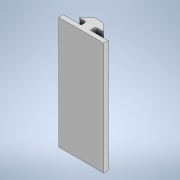
# Autodesk Inventor part: ZItemSpacer
Saved by Autodesk Inventor 2020 (Build 240168000, 168)
## iProperties
Created: 2022-06-06
Part Number: ZItemSpacer
Material: Ogólny
Document SubType Name: Modeling
Designer: mikoma
Density: 1 g/cm^3
Appearance: Domyślna
Author: mikoma
Autodesk Inventor part; units mm, degrees
ref_plane "YZ Plane" through (0, 0, 0) normal (1, 0, 0) x (0, 1, 0)
ref_plane "XZ Plane" through (0, 0, 0) normal (0, 1, 0) x (-1, 0, 0)
ref_plane "XY Plane" through (0, 0, 0) normal (0, 0, 1) x (1, 0, 0)
sketch "Szkic1" plane through (0, 0, 0) normal (0, 1, 0) x (-1, 0, 0)
  arc A0 (11.3, 0) -> (10.5, -0.8) centre (11.3, -0.8) ccw
  line L0 (10.5, -0.8) -> (10.5, -1.5)
  arc A1 (10.5, -1.5) -> (10.8, -1.8) centre (10.8, -1.5) ccw
  line L1 (10.8, -1.8) -> (12.9176, -1.8)
  arc A2 (13.5062, -3.221) -> (12.9176, -1.8) centre (12.9176, -2.6324) ccw
  line L2 (13.5062, -3.221) -> (11.2559, -5.4713)
  arc A3 (9.1346, -6.35) -> (11.2559, -5.4713) centre (9.1346, -3.35) ccw
  line L3 (9.1346, -6.35) -> (6.8654, -6.35)
  arc A4 (4.7441, -5.4713) -> (6.8654, -6.35) centre (6.8654, -3.35) ccw
  line L4 (4.7441, -5.4713) -> (2.4938, -3.221)
  arc A5 (3.0824, -1.8) -> (2.4938, -3.221) centre (3.0824, -2.6324) ccw
  line L5 (3.0824, -1.8) -> (5.2, -1.8)
  arc A6 (5.2, -1.8) -> (5.5, -1.5) centre (5.2, -1.5) ccw
  line L6 (5.5, -1.5) -> (5.5, -0.8)
  arc A7 (5.5, -0.8) -> (4.7, 0) centre (4.7, -0.8) ccw
  line L7 (0, 0) -> (4.7, 0)
  arc A8 (0, 0) -> (-2, -2) centre (0, -2) ccw
  line L8 (-2, -6.7) -> (-2, -2)
  arc A9 (-2, -6.7) -> (-1.2, -7.5) centre (-1.2, -6.7) ccw
  line L9 (-1.2, -7.5) -> (-0.5, -7.5)
  arc A10 (-0.5, -7.5) -> (-0.2, -7.2) centre (-0.5, -7.2) ccw
  line L10 (-0.2, -7.2) -> (-0.2, -5.0824)
  arc A11 (1.221, -4.4938) -> (-0.2, -5.0824) centre (0.6324, -5.0824) ccw
  line L11 (1.221, -4.4938) -> (3.4713, -6.7441)
  arc A12 (4.35, -8.8654) -> (3.4713, -6.7441) centre (1.35, -8.8654) ccw
  line L12 (4.35, -8.8654) -> (4.35, -11.1346)
  arc A13 (3.4713, -13.2559) -> (4.35, -11.1346) centre (1.35, -11.1346) ccw
  line L13 (3.4713, -13.2559) -> (1.221, -15.5062)
  arc A14 (-0.2, -14.9176) -> (1.221, -15.5062) centre (0.6324, -14.9176) ccw
  line L14 (-0.2, -14.9176) -> (-0.2, -12.8)
  arc A15 (-0.2, -12.8) -> (-0.5, -12.5) centre (-0.5, -12.8) ccw
  line L15 (-0.5, -12.5) -> (-1.2, -12.5)
  arc A16 (-1.2, -12.5) -> (-2, -13.3) centre (-1.2, -13.3) ccw
  line L16 (-2, -18) -> (-2, -13.3)
  arc A17 (-2, -18) -> (0, -20) centre (0, -18) ccw
  line L17 (4.7, -20) -> (0, -20)
  arc A18 (4.7, -20) -> (5.5, -19.2) centre (4.7, -19.2) ccw
  line L18 (5.5, -19.2) -> (5.5, -18.5)
  arc A19 (5.5, -18.5) -> (5.2, -18.2) centre (5.2, -18.5) ccw
  line L19 (5.2, -18.2) -> (3.0824, -18.2)
  arc A20 (2.4938, -16.779) -> (3.0824, -18.2) centre (3.0824, -17.3676) ccw
  line L20 (2.4938, -16.779) -> (4.7441, -14.5287)
  arc A21 (6.8654, -13.65) -> (4.7441, -14.5287) centre (6.8654, -16.65) ccw
  line L21 (6.8654, -13.65) -> (9.1346, -13.65)
  arc A22 (11.2559, -14.5287) -> (9.1346, -13.65) centre (9.1346, -16.65) ccw
  line L22 (11.2559, -14.5287) -> (13.5062, -16.779)
  arc A23 (12.9176, -18.2) -> (13.5062, -16.779) centre (12.9176, -17.3676) ccw
  line L23 (12.9176, -18.2) -> (10.8, -18.2)
  arc A24 (10.8, -18.2) -> (10.5, -18.5) centre (10.8, -18.5) ccw
  line L24 (10.5, -18.5) -> (10.5, -19.2)
  arc A25 (10.5, -19.2) -> (11.3, -20) centre (11.3, -19.2) ccw
  line L25 (16, -20) -> (11.3, -20)
  arc A26 (16, -20) -> (18, -18) centre (16, -18) ccw
  line L26 (18, -13.3) -> (18, -18)
  arc A27 (18, -13.3) -> (17.2, -12.5) centre (17.2, -13.3) ccw
  line L27 (17.2, -12.5) -> (16.5, -12.5)
  arc A28 (16.5, -12.5) -> (16.2, -12.8) centre (16.5, -12.8) ccw
  line L28 (16.2, -12.8) -> (16.2, -14.9176)
  arc A29 (14.779, -15.5062) -> (16.2, -14.9176) centre (15.3676, -14.9176) ccw
  line L29 (14.779, -15.5062) -> (12.5287, -13.2559)
  arc A30 (11.65, -11.1346) -> (12.5287, -13.2559) centre (14.65, -11.1346) ccw
  line L30 (11.65, -11.1346) -> (11.65, -8.8654)
  arc A31 (12.5287, -6.7441) -> (11.65, -8.8654) centre (14.65, -8.8654) ccw
  line L31 (12.5287, -6.7441) -> (14.779, -4.4938)
  arc A32 (16.2, -5.0824) -> (14.779, -4.4938) centre (15.3676, -5.0824) ccw
  line L32 (16.2, -5.0824) -> (16.2, -7.2)
  arc A33 (16.2, -7.2) -> (16.5, -7.5) centre (16.5, -7.2) ccw
  line L33 (16.5, -7.5) -> (17.2, -7.5)
  arc A34 (17.2, -7.5) -> (18, -6.7) centre (17.2, -6.7) ccw
  line L34 (18, -2) -> (18, -6.7)
  arc A35 (18, -2) -> (16, 0) centre (16, -2) ccw
  line L35 (11.3, 0) -> (16, 0)
  circle A36 centre (8, -10) radius 2.15
  line L36 (18, 2) -> (-2, 2)
  line L37 (-2, 2) -> (-2, 0)
  line L38 (-2, 0) -> (18, 0)
  line L39 (18, 0) -> (18, 2)
  line L40 (10.5, -1.8) -> (5.5, -1.8)
  line L41 (5.5, -1.8) -> (5.5, 0)
  line L42 (5.5, 0) -> (10.5, 0)
  line L43 (10.5, 0) -> (10.5, -1.8)
  point P0 (0, 0)
  point P1 (16, 0)
  point P2 (4.7, 0)
  dimension "d0" = 2
  constraints: 88 end point, 72 point on circle, 37 centre point, 10 horizontal, 8 vertical, 4 parallel, 4 point on line, 3 collinear, 2 perpendicular, 168 other
  measures "d0" distance of L38.end L36.start
extrude "Wyciągnięcie proste1" add sketch "Szkic1" along normal blind 50 contours L38 L7 L37 L36 L39 L35 | L0 L43 L40 L41 L6 L38 | A1 L1 A2 L2 A3 L3 A4 L4 A5 L5 A6 L41 L40 L43
thicken "Pogrubienie1" operation add thickness 0.5 both sides no extend neighbours yes toward (-1, 0, 0) faces at (-5.5, 16.6667, -1.0333) (-5.4479, 33.3333, -1.669) (-4.4941, 16.6667, -1.8) (-2.4938, 33.3333, -2.0438) (-3.2439, 16.6667, -3.9711) (-5.5386, 33.3333, -6.0406) (-7.6218, 16.6667, -6.35) (-10.6346, 33.3333, -5.9481) (-12.006, 16.6667, -4.7212) (-13.1748, 33.3333, -1.8407) (-12.2117, 16.6667, -1.8) (-10.5402, 33.3333, -1.65) (-10.5, 16.6667, -1.2667)
